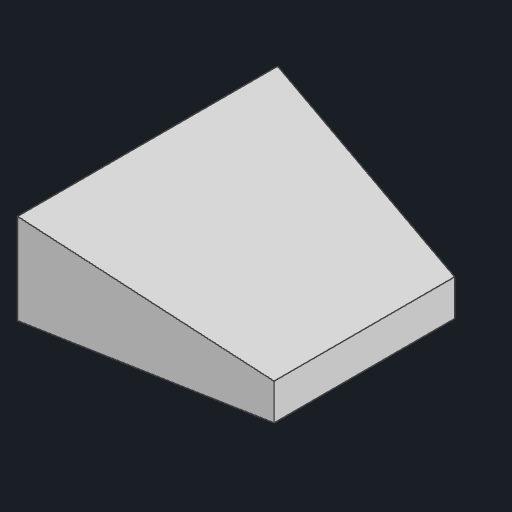
# Autodesk Inventor part: finger
Saved by Autodesk Inventor 2023 (Build 270158000, 158)
## iProperties
Created: 2024-02-21
Part Number: finger
Material: Generic
Document SubType Name: Modeling
Designer: valer
Density: 1 g/cm^3
Appearance: Default
Author: valer
Autodesk Inventor part; units mm, degrees
ref_plane "YZ Plane" through (0, 0, 0) normal (1, 0, 0) x (0, 1, 0)
ref_plane "XZ Plane" through (0, 0, 0) normal (0, 1, 0) x (-1, 0, 0)
ref_plane "XY Plane" through (0, 0, 0) normal (0, 0, 1) x (1, 0, 0)
sketch "Sketch1" plane through (0, 0, 0) normal (0, 0, 1) x (1, 0, 0)
  line L0 (100, 62.5) -> (250, 25)
  line L1 (250, 25) -> (250, 0)
  line L2 (250, 0) -> (100, 0)
  line L3 (100, 0) -> (100, 62.5)
  line L4 (-50, 0) -> (300, 0) construction
  point P0 (0, 0)
  dimension "d0" = 62.5
  dimension "d1" = 150
  dimension "d2" = 25
  dimension "d8" = 100
  constraints: 8 end point, 2 perpendicular, 1 collinear, 1 horizontal
  measures "d0" distance of L2.end L0.start
  measures "d1" distance of L1.end L2.end
  measures "d2" distance of L0.end L1.end
  measures "d8" distance from line of L3 point (0, 0)
extrude "Extrusion1" add sketch "Sketch1" along normal mid plane 180
sketch "Sketch2" plane through (100, 0, 90) normal (0, -1, 0) x (1, 0, 0)
  line L0 (150, -180) -> (150, 0) projected
  line L1 (0, 0) -> (150, 0) projected
  line L2 (0, 0) -> (0, -180) projected
  line L3 (150, -180) -> (0, -180) projected
  line L4 (0, 0) -> (150, -27.5)
  line L5 (0, -180) -> (0, 0) projected
  line L6 (0, -90) -> (150, -90) construction
  line L7 (0, -180) -> (150, -152.5)
  point P0 (-100, -90)
  point P1 (150, -152.5)
  dimension "d5" = 62.5
  constraints: 6 end point, 2 midpoint, 1 point on line, 1 symmetric about line
  measures "d5" distance from line of L6 L4.end
extrude "Extrusion2" cut sketch "Sketch2" against normal through all contours L3 L7 L0 | L4 L1 L0
body "Solid1"
